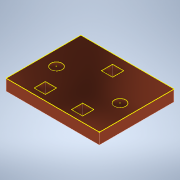
# Autodesk Inventor part: motorbase_3
Saved by Autodesk Inventor 2022 (Build 260153000, 153)
## iProperties
Created: 2023-04-18
Part Number: motorbase_3
Material: 一般
Document SubType Name: Modeling
Designer: Johnny Jou
Density: 1 g/cm^3
Appearance: 銅 - 拋光
Author: Johnny Jou
Autodesk Inventor part; units mm, degrees
ref_plane "YZ Plane" through (0, 0, 0) normal (1, 0, 0) x (0, 1, 0)
ref_plane "XZ Plane" through (0, 0, 0) normal (0, 1, 0) x (-1, 0, 0)
ref_plane "XY Plane" through (0, 0, 0) normal (0, 0, 1) x (1, 0, 0)
sketch "草圖1" plane through (0, 0, 0) normal (0, 1, 0) x (-1, 0, 0)
  line L0 (25, 0) -> (0, 0)
  line L1 (0, 0) -> (0, -20)
  line L2 (0, -20) -> (25, -20)
  line L3 (25, -20) -> (25, 0)
  line L4 (6.5, -14.5) -> (18.5, -14.5) construction
  line L5 (5.5, -17.5) -> (8.5, -17.5)
  line L6 (8.5, -17.5) -> (8.5, -14.5)
  line L7 (8.5, -14.5) -> (5.5, -14.5)
  line L8 (5.5, -14.5) -> (5.5, -17.5)
  line L9 (9, -4.5) -> (16, -4.5) construction
  line L10 (9, -4.5) -> (6, -4.5)
  line L11 (6, -4.5) -> (6, -1.5)
  line L12 (6, -1.5) -> (9, -1.5)
  line L13 (9, -1.5) -> (9, -4.5)
  line L14 (16, -4.5) -> (19, -4.5)
  line L15 (19, -4.5) -> (19, -1.5)
  line L16 (19, -1.5) -> (16, -1.5)
  line L17 (16, -1.5) -> (16, -4.5)
  line L18 (16.5, -17.5) -> (19.5, -17.5)
  line L19 (19.5, -17.5) -> (19.5, -14.5)
  line L20 (19.5, -14.5) -> (16.5, -14.5)
  line L21 (16.5, -14.5) -> (16.5, -17.5)
  circle A0 centre (4, -9.5) radius 1.5
  circle A1 centre (21, -9.5) radius 1.5
  line L22 (11, -14.5) -> (14, -14.5)
  line L23 (14, -14.5) -> (14, -17.5)
  line L24 (14, -17.5) -> (11, -17.5)
  line L25 (11, -17.5) -> (11, -14.5)
  point P0 (19, 16.3854)
  point P1 (12.5, -17.5)
  point P2 (12.5, -14.5)
  dimension "d0" = 25
  dimension "d1" = 20
  dimension "d2" = 3
  dimension "d3" = 3
  dimension "d4" = 0
  dimension "d5" = 10
  dimension "d6" = 3
  dimension "d7" = 3
  dimension "d8" = 3
  dimension "d9" = 3
  dimension "d10" = 3
  dimension "d11" = 3
  dimension "d12" = 3
  dimension "d13" = 5
  dimension "d14" = 5
  dimension "d15" = 8
  dimension "d16" = 2.5
  dimension "d18" = 7
  dimension "d22" = 5.5
  dimension "d23" = 5.5
  dimension "d24" = 6
  dimension "d25" = 3
  dimension "d26" = 3
  constraints: 52 end point, 12 parallel, 7 horizontal, 6 perpendicular, 2 centre point, 2 collinear, 2 midpoint, 2 point on line, 1 coincident, 1 vertical alignment
  measures "d0" distance of L1.end L2.end
  measures "d1" distance of L2.end L0.start
  measures "d2" distance of L7.end L5.start
  measures "d3" distance of L6.end L7.end
  measures "d4" distance between parallel lines of L4 L7
  measures "d5" distance between parallel lines of L4 L9
  measures "d6" distance of L11.start L12.start
  measures "d7" distance of L12.start L13.start
  measures "d8" distance of L21.end L18.end
  measures "d9" distance of L18.end L20.start
  measures "d10" distance of L9.end L14.end
  measures "d11" diameter of A0
  measures "d12" diameter of A1
  measures "d13" distance from line of L10 A0.centre
  measures "d14" distance from line of L14 A1.centre
  measures "d15" distance between parallel lines of L21 L6
  measures "d16" distance between parallel lines of L2 L18
  measures "d18" distance between parallel lines of L13 L17
  measures "d22" distance between parallel lines of L3 L19
  measures "d23" distance between parallel lines of L1 L8
  measures "d24" distance between parallel lines of L3 L15
  measures "d25" distance of L22.end L23.end
  measures "d26" distance of L23.end L24.end
extrude "擠出1" add sketch "草圖1" along normal blind 3 contours L3 L2 L1 L0 | L8 L7 L6 L5 | L21 L20 L19 L18
sketch "草圖2" plane through (0, 3, 0) normal (0, 1, 0) x (1, 0, 0)
  line L0 (0, 0) -> (0, 20) projected
  line L1 (0, 20) -> (-25, 20) projected
  line L2 (-25, 20) -> (-25, 0) projected
  line L3 (-25, 0) -> (0, 0) projected
  circle A0 centre (-21, 9.5) radius 1.5 projected
  circle A1 centre (-4, 9.5) radius 1.5 projected
  line L4 (-11, 14.5) -> (-14, 14.5) projected
  line L5 (-14, 14.5) -> (-14, 17.5) projected
  line L6 (-14, 17.5) -> (-11, 17.5) projected
  line L7 (-11, 17.5) -> (-11, 14.5) projected
  line L8 (-9, 1.5) -> (-9, 4.5) projected
  line L9 (-9, 4.5) -> (-6, 4.5) projected
  line L10 (-6, 4.5) -> (-6, 1.5) projected
  line L11 (-6, 1.5) -> (-9, 1.5) projected
  line L12 (-16, 4.5) -> (-16, 1.5) projected
  line L13 (-16, 1.5) -> (-19, 1.5) projected
  line L14 (-19, 1.5) -> (-19, 4.5) projected
  line L15 (-19, 4.5) -> (-16, 4.5) projected
